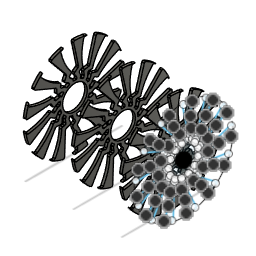
knobs + spokes v4 (Autodesk Fusion 360 archive; units mm, degrees)
design "spoke support"
Autodesk Fusion 360 part; units mm, degrees
sketch "Sketch1" plane through (0, 0, 0) normal (1, 0, 0) x (0, 0, -1)
  circle A0 centre (0, 0) radius 5
  circle A1 centre (0, 0) radius 20 construction
  circle A2 centre (0, 0) radius 6
  line L0 (-0.021, 20) -> (-0.0893, 19.9864)
  line L1 (-0.481, 19.3928) -> (1.4345, 10.3121)
  line L2 (1.2453, 9.8089) -> (-0.1, 8.8)
  line L3 (-0.2, 8.1) -> (0.71, 6.8867)
  line L4 (0.75, 6.7667) -> (0.75, 5.9529)
  arc A3 (-0.0893, 19.9864) -> (-0.481, 19.3928) centre (0.0083, 19.496) ccw
  arc A4 (1.2453, 9.8089) -> (1.4345, 10.3121) centre (0.9453, 10.2089) ccw
  arc A5 (-0.1, 8.8) -> (-0.2, 8.1) centre (0.2, 8.4) ccw
  arc A6 (0.75, 6.7667) -> (0.71, 6.8867) centre (0.55, 6.7667) ccw
  line L5 (4.9442, 19.3792) -> (4.0475, 19.3979)
  arc A7 (4.0475, 19.3979) -> (3.5372, 18.9052) centre (4.0371, 18.898) ccw
  arc A8 (2.9152, 8.8921) -> (3.1386, 9.6333) centre (2.7238, 9.3541) ccw
  line L6 (2.9152, 8.8921) -> (2.0875, 8.5494)
  arc A9 (2.0875, 8.5494) -> (1.8169, 7.8961) centre (2.2789, 8.0874) ccw
  line L7 (1.8169, 7.8961) -> (2.3972, 6.4949)
  arc A10 (2.4062, 6.3687) -> (2.3972, 6.4949) centre (2.2124, 6.4184) ccw
  line L8 (2.4062, 6.3687) -> (2.2042, 5.5805)
  spline S0 degree 5 poles (3.5372, 18.9052) (3.4914, 18.7092) (3.403, 18.318) (3.2802, 17.7339) (3.1365, 16.9608) (2.9923, 16.0043) (2.887, 15.0588) (2.8238, 14.1251) (2.8051, 13.2038) (2.8293, 12.2946) (2.8936, 11.3966) (2.9744, 10.6864) (3.0506, 10.1582) (3.1082, 9.8079) (3.1386, 9.6333) knots 0 0 0 0 0 0 0.1 0.2 0.3 0.4 0.5 0.6 0.7 0.8 0.9 1 1 1 1 1 1
  arc A11 (4.9442, 19.3792) -> (-0.021, 20) centre (0, 0) ccw
  line L9 (-2.4805, 6.3401) -> (-2.1024, 5.6196)
  arc A12 (-2.4805, 6.3401) -> (-2.5717, 6.4278) centre (-2.6576, 6.2472) ccw
  line L10 (-3.9413, 7.0792) -> (-2.5717, 6.4278)
  arc A13 (-4.1781, 7.7455) -> (-3.9413, 7.0792) centre (-3.7265, 7.5308) ccw
  line L11 (-3.4558, 9.264) -> (-4.1781, 7.7455)
  arc A14 (-3.4558, 9.264) -> (-3.5221, 9.7975) centre (-3.9073, 9.4788) ccw
  line L12 (-9.4382, 16.948) -> (-3.5221, 9.7975)
  arc A15 (-9.3672, 17.6555) -> (-9.4382, 16.948) centre (-9.0529, 17.2667) ccw
  line L13 (-9.313, 17.6994) -> (-9.3672, 17.6555)
  arc A16 (-4.6281, 19.4571) -> (-9.313, 17.6994) centre (0, 0) ccw
  line L14 (-4.6281, 19.4571) -> (-5.4307, 19.057)
  arc A17 (-5.4307, 19.057) -> (-5.6537, 18.3836) centre (-5.2076, 18.6095) ccw
  arc A18 (-1.5511, 9.2283) -> (-1.6977, 9.9884) centre (-1.9352, 9.5485) ccw
  line L15 (-1.5511, 9.2283) -> (-2.1247, 8.5402)
  arc A19 (-2.1247, 8.5402) -> (-2.0607, 7.836) centre (-1.7406, 8.2201) ccw
  line L16 (-2.0607, 7.836) -> (-0.8957, 6.865)
  arc A20 (-0.8291, 6.7574) -> (-0.8957, 6.865) centre (-1.0237, 6.7114) ccw
  line L17 (-0.8291, 6.7574) -> (-0.6417, 5.9656)
  spline S1 degree 5 poles (-5.6537, 18.3836) (-5.6031, 18.1887) (-5.4996, 17.8012) (-5.3369, 17.227) (-5.1049, 16.4756) (-4.788, 15.5617) (-4.4419, 14.6755) (-4.0639, 13.8194) (-3.6523, 12.9949) (-3.2083, 12.2011) (-2.7341, 11.4359) (-2.3325, 10.8446) (-2.0196, 10.4123) (-1.8058, 10.1289) (-1.6977, 9.9884) knots 0 0 0 0 0 0 0.1 0.2 0.3 0.4 0.5 0.6 0.7 0.8 0.9 1 1 1 1 1 1
  line L18 (-5.1428, 4.4611) -> (-4.4731, 3.9989)
  arc A21 (-5.1428, 4.4611) -> (-5.2643, 4.4964) centre (-5.2564, 4.2965) ccw
  line L19 (-6.7797, 4.4367) -> (-5.2643, 4.4964)
  arc A22 (-7.299, 4.9167) -> (-6.7797, 4.4367) centre (-6.7994, 4.9363) ccw
  line L20 (-7.3652, 6.5969) -> (-7.299, 4.9167)
  arc A23 (-7.3652, 6.5969) -> (-7.6718, 7.0385) centre (-7.8648, 6.5772) ccw
  line L21 (-16.2332, 10.6205) -> (-7.6718, 7.0385)
  arc A24 (-16.4992, 11.28) -> (-16.2332, 10.6205) centre (-16.0402, 11.0818) ccw
  line L22 (-16.4716, 11.344) -> (-16.4992, 11.28)
  arc A25 (-13.1402, 15.0777) -> (-16.4716, 11.344) centre (0, 0) ccw
  line L23 (-13.1402, 15.0777) -> (-13.6649, 14.3503)
  arc A26 (-13.6649, 14.3503) -> (-13.5494, 13.6505) centre (-13.2594, 14.0578) ccw
  arc A27 (-5.6621, 7.4504) -> (-6.1451, 8.0554) centre (-6.1509, 7.5554) ccw
  line L24 (-5.6621, 7.4504) -> (-5.8501, 6.5746)
  arc A28 (-5.8501, 6.5746) -> (-5.4662, 5.9808) centre (-5.3613, 6.4696) ccw
  line L25 (-5.4662, 5.9808) -> (-3.9834, 5.6624)
  arc A29 (-3.8745, 5.5981) -> (-3.9834, 5.6624) centre (-4.0254, 5.4669) ccw
  line L26 (-3.8745, 5.5981) -> (-3.3405, 4.9841)
  spline S2 degree 5 poles (-13.5494, 13.6505) (-13.414, 13.5014) (-13.1423, 13.2064) (-12.7314, 12.7736) (-12.1768, 12.2161) (-11.4715, 11.5541) (-10.7531, 10.9303) (-10.0206, 10.3479) (-9.273, 9.8091) (-8.511, 9.3126) (-7.7354, 8.8553) (-7.1051, 8.5185) (-6.6271, 8.2811) (-6.3061, 8.1295) (-6.1451, 8.0554) knots 0 0 0 0 0 0 0.1 0.2 0.3 0.4 0.5 0.6 0.7 0.8 0.9 1 1 1 1 1 1
  line L27 (-6.6269, 1.5602) -> (-5.8191, 1.4621)
  arc A30 (-6.6269, 1.5602) -> (-6.7509, 1.5349) centre (-6.651, 1.3616) ccw
  line L28 (-8.065, 0.7778) -> (-6.7509, 1.5349)
  arc A31 (-8.7478, 0.9615) -> (-8.065, 0.7778) centre (-8.3146, 1.2111) ccw
  line L29 (-9.5873, 2.4185) -> (-8.7478, 0.9615)
  arc A32 (-9.5873, 2.4185) -> (-10.064, 2.667) centre (-10.0205, 2.1689) ccw
  line L30 (-19.3094, 1.8601) -> (-10.064, 2.667)
  arc A33 (-19.8514, 2.3204) -> (-19.3094, 1.8601) centre (-19.3529, 2.3582) ccw
  line L31 (-19.8567, 2.3899) -> (-19.8514, 2.3204)
  arc A34 (-18.642, 7.2441) -> (-19.8567, 2.3899) centre (0, 0) ccw
  line L32 (-18.642, 7.2441) -> (-18.7686, 6.3562)
  arc A35 (-18.7686, 6.3562) -> (-18.341, 5.7902) centre (-18.2736, 6.2856) ccw
  arc A36 (-8.4759, 3.9657) -> (-9.1847, 4.2769) centre (-8.9576, 3.8315) ccw
  line L33 (-8.4759, 3.9657) -> (-8.2354, 3.1028)
  arc A37 (-8.2354, 3.1028) -> (-7.6195, 2.7554) centre (-7.7538, 3.2371) ccw
  line L34 (-7.6195, 2.7554) -> (-6.1586, 3.1626)
  arc A38 (-6.0323, 3.1563) -> (-6.1586, 3.1626) centre (-6.1049, 2.97) ccw
  line L35 (-6.0323, 3.1563) -> (-5.2741, 2.8608)
  spline S3 degree 5 poles (-18.341, 5.7902) (-18.1519, 5.721) (-17.7742, 5.5862) (-17.2092, 5.3939) (-16.4591, 5.158) (-15.527, 4.8996) (-14.601, 4.6811) (-13.6817, 4.5058) (-12.7694, 4.3761) (-11.8639, 4.2906) (-10.9647, 4.2462) (-10.25, 4.2408) (-9.7164, 4.2528) (-9.3617, 4.2677) (-9.1847, 4.2769) knots 0 0 0 0 0 0 0.1 0.2 0.3 0.4 0.5 0.6 0.7 0.8 0.9 1 1 1 1 1 1
  line L36 (-6.5929, -1.6982) -> (-5.832, -1.4097)
  arc A39 (-6.5929, -1.6982) -> (-6.6909, -1.7782) centre (-6.522, -1.8852) ccw
  line L37 (-7.5027, -3.0593) -> (-6.6909, -1.7782)
  arc A40 (-8.1927, -3.214) -> (-7.5027, -3.0593) centre (-7.925, -2.7916) ccw
  line L38 (-9.613, -2.3139) -> (-8.1927, -3.214)
  arc A41 (-9.613, -2.3139) -> (-10.1506, -2.3154) centre (-9.8807, -2.7363) ccw
  line L39 (-17.962, -7.3265) -> (-10.1506, -2.3154)
  arc A42 (-18.6559, -7.1708) -> (-17.962, -7.3265) centre (-18.232, -6.9056) ccw
  line L40 (-18.6929, -7.1117) -> (-18.6559, -7.1708)
  arc A43 (-19.8731, -2.2491) -> (-18.6929, -7.1117) centre (0, 0) ccw
  line L41 (-19.8731, -2.2491) -> (-19.5726, -3.0941)
  arc A44 (-19.5726, -3.0941) -> (-18.931, -3.3966) centre (-19.1015, -2.9265) ccw
  arc A45 (-9.348, -0.4275) -> (-10.1202, -0.4813) centre (-9.7121, -0.7702) ccw
  line L42 (-9.348, -0.4275) -> (-8.734, -1.0798)
  arc A46 (-8.734, -1.0798) -> (-8.0273, -1.1012) centre (-8.37, -0.7371) ccw
  line L43 (-8.0273, -1.1012) -> (-6.9229, -0.0617)
  arc A47 (-6.8081, -0.0086) -> (-6.9229, -0.0617) centre (-6.7858, -0.2073) ccw
  line L44 (-6.8081, -0.0086) -> (-5.9994, 0.0821)
  spline S4 degree 5 poles (-18.931, -3.3966) (-18.7314, -3.3699) (-18.3343, -3.3138) (-17.7447, -3.2215) (-16.9708, -3.0817) (-16.0254, -2.8774) (-15.1039, -2.6405) (-14.2085, -2.3685) (-13.3404, -2.0593) (-12.4989, -1.7142) (-11.682, -1.3357) (-11.0467, -1.0083) (-10.5798, -0.7498) (-10.2727, -0.5718) (-10.1202, -0.4813) knots 0 0 0 0 0 0 0.1 0.2 0.3 0.4 0.5 0.6 0.7 0.8 0.9 1 1 1 1 1 1
  line L45 (-5.0485, -4.5676) -> (-4.5089, -3.9585)
  arc A48 (-5.0485, -4.5676) -> (-5.0981, -4.6839) centre (-4.8988, -4.7002) ccw
  line L46 (-5.2216, -6.1955) -> (-5.0981, -4.6839)
  arc A49 (-5.7606, -6.6532) -> (-5.2216, -6.1955) centre (-5.7199, -6.1548) ccw
  line L47 (-7.4366, -6.5163) -> (-5.7606, -6.6532)
  arc A50 (-7.4366, -6.5163) -> (-7.9119, -6.7675) centre (-7.4773, -7.0146) ccw
  line L48 (-12.4998, -14.8347) -> (-7.9119, -6.7675)
  arc A51 (-13.1865, -15.0193) -> (-12.4998, -14.8347) centre (-12.9344, -14.5875) ccw
  line L49 (-13.2468, -14.9841) -> (-13.1865, -15.0193)
  arc A52 (-16.5516, -11.227) -> (-13.2468, -14.9841) centre (0, 0) ccw
  line L50 (-16.5516, -11.227) -> (-15.8928, -11.8355)
  arc A53 (-15.8928, -11.8355) -> (-15.1841, -11.8052) centre (-15.5535, -11.4682) ccw
  arc A54 (-8.0786, -4.7227) -> (-8.7373, -5.1293) centre (-8.2417, -5.1954) ccw
  line L51 (-8.0786, -4.7227) -> (-7.2318, -5.015)
  arc A55 (-7.2318, -5.015) -> (-6.596, -4.7055) centre (-7.0687, -4.5424) ccw
  line L52 (-6.596, -4.7055) -> (-6.1013, -3.2718)
  arc A56 (-6.0243, -3.1715) -> (-6.1013, -3.2718) centre (-5.9122, -3.3371) ccw
  line L53 (-6.0243, -3.1715) -> (-5.3504, -2.7154)
  spline S5 degree 5 poles (-15.1841, -11.8052) (-15.0198, -11.6888) (-14.6942, -11.4546) (-14.215, -11.0989) (-13.5948, -10.6155) (-12.8526, -9.9952) (-12.1468, -9.3572) (-11.4803, -8.7002) (-10.8553, -8.0231) (-10.2706, -7.3264) (-9.7232, -6.6117) (-9.3128, -6.0265) (-9.0195, -5.5806) (-8.8303, -5.2802) (-8.7373, -5.1293) knots 0 0 0 0 0 0 0.1 0.2 0.3 0.4 0.5 0.6 0.7 0.8 0.9 1 1 1 1 1 1
  line L54 (-2.3476, -6.3906) -> (-2.1528, -5.6005)
  arc A57 (-2.3476, -6.3906) -> (-2.3375, -6.5166) centre (-2.1534, -6.4384) ccw
  line L55 (-1.7443, -7.9124) -> (-2.3375, -6.5166)
  arc A58 (-2.0089, -8.5682) -> (-1.7443, -7.9124) centre (-2.2045, -8.108) ccw
  line L56 (-3.5565, -9.2258) -> (-2.0089, -8.5682)
  arc A59 (-3.5565, -9.2258) -> (-3.8606, -9.6691) centre (-3.3609, -9.686) ccw
  line L57 (-4.174, -18.9444) -> (-3.8606, -9.6691)
  arc A60 (-4.6963, -19.427) -> (-4.174, -18.9444) centre (-4.6737, -18.9275) ccw
  line L58 (-4.766, -19.4238) -> (-4.6963, -19.427)
  arc A61 (-9.4383, -17.6329) -> (-4.766, -19.4238) centre (0, 0) ccw
  line L59 (-9.4383, -17.6329) -> (-8.5721, -17.8656)
  arc A62 (-8.5721, -17.8656) -> (-7.9587, -17.5094) centre (-8.4424, -17.3827) ccw
  arc A63 (-4.9585, -7.9361) -> (-5.3528, -8.6022) centre (-4.8833, -8.4304) ccw
  line L60 (-4.9585, -7.9361) -> (-4.0729, -7.8014)
  arc A64 (-4.0729, -7.8014) -> (-3.6538, -7.2318) centre (-4.1481, -7.307) ccw
  line L61 (-3.6538, -7.2318) -> (-3.8819, -5.7325)
  arc A65 (-3.8604, -5.6078) -> (-3.8819, -5.7325) centre (-3.6842, -5.7024) ccw
  line L62 (-3.8604, -5.6078) -> (-3.4756, -4.8908)
  spline S6 degree 5 poles (-7.9587, -17.5094) (-7.8673, -17.33) (-7.6879, -16.9713) (-7.4289, -16.4336) (-7.1043, -15.7173) (-6.7354, -14.8232) (-6.4069, -13.9303) (-6.1221, -13.0388) (-5.8834, -12.1488) (-5.6894, -11.2602) (-5.5369, -10.3729) (-5.4454, -9.6641) (-5.393, -9.1329) (-5.365, -8.7791) (-5.3528, -8.6022) knots 0 0 0 0 0 0 0.1 0.2 0.3 0.4 0.5 0.6 0.7 0.8 0.9 1 1 1 1 1 1
  line L63 (0.8912, -6.7495) -> (0.6964, -5.9594)
  arc A66 (0.8912, -6.7495) -> (0.9587, -6.8565) centre (1.0854, -6.7017) ccw
  line L64 (2.1326, -7.8167) -> (0.9587, -6.8565)
  arc A67 (2.203, -8.5203) -> (2.1326, -7.8167) centre (1.816, -8.2037) ccw
  line L65 (1.1383, -9.8219) -> (2.203, -8.5203)
  arc A68 (1.1383, -9.8219) -> (1.075, -10.3557) centre (1.5254, -10.1384) ccw
  line L66 (5.108, -18.7142) -> (1.075, -10.3557)
  arc A69 (4.8698, -19.3842) -> (5.108, -18.7142) centre (4.6577, -18.9315) ccw
  line L67 (4.8067, -19.4138) -> (4.8698, -19.3842)
  arc A70 (-0.1628, -19.9993) -> (4.8067, -19.4138) centre (0, 0) ccw
  line L68 (-0.1628, -19.9993) -> (0.7123, -19.8029)
  arc A71 (0.7123, -19.8029) -> (1.0899, -19.2024) centre (0.6028, -19.315) ccw
  arc A72 (-0.7024, -9.3314) -> (-0.742, -10.1045) centre (-0.4061, -9.7341) ccw
  line L69 (-0.7024, -9.3314) -> (0.0191, -8.8005)
  arc A73 (0.0191, -8.8005) -> (0.1255, -8.1015) centre (-0.2772, -8.3978) ccw
  line L70 (0.1255, -8.1015) -> (-0.7732, -6.8799)
  arc A74 (-0.8121, -6.7595) -> (-0.7732, -6.8799) centre (-0.6121, -6.7613) ccw
  line L71 (-0.8121, -6.7595) -> (-0.8047, -5.9458)
  spline S7 degree 5 poles (1.0899, -19.2024) (1.0875, -19.0011) (1.0797, -18.6001) (1.0591, -18.0036) (1.0137, -17.2185) (0.9247, -16.2554) (0.8007, -15.3121) (0.6386, -14.3904) (0.4363, -13.4914) (0.1952, -12.6144) (-0.0821, -11.7579) (-0.3306, -11.0877) (-0.5309, -10.593) (-0.6707, -10.2667) (-0.742, -10.1045) knots 0 0 0 0 0 0 0.1 0.2 0.3 0.4 0.5 0.6 0.7 0.8 0.9 1 1 1 1 1 1
  line L72 (3.9257, -5.5623) -> (3.3861, -4.9532)
  arc A75 (3.9257, -5.5623) -> (4.0353, -5.6256) centre (4.0755, -5.4296) ccw
  line L73 (5.5209, -5.9303) -> (4.0353, -5.6256)
  arc A76 (5.9103, -6.5206) -> (5.5209, -5.9303) centre (5.4205, -6.4201) ccw
  line L74 (5.5724, -8.1678) -> (5.9103, -6.5206)
  arc A77 (5.5724, -8.1678) -> (5.7644, -8.6699) centre (6.0622, -8.2683) ccw
  line L75 (13.2198, -14.1968) -> (5.7644, -8.6699)
  arc A78 (13.3203, -14.9008) -> (13.2198, -14.1968) centre (12.922, -14.5984) ccw
  line L76 (13.2781, -14.9563) -> (13.3203, -14.9008)
  arc A79 (9.15, -17.7842) -> (13.2781, -14.9563) centre (0, 0) ccw
  line L77 (9.15, -17.7842) -> (9.8336, -17.2035)
  arc A80 (9.8336, -17.2035) -> (9.8889, -16.4964) centre (9.5098, -16.8225) ccw
  arc A81 (3.7145, -8.589) -> (4.0387, -9.2919) centre (4.1641, -8.8079) ccw
  line L78 (3.7145, -8.589) -> (4.1067, -7.7836)
  arc A82 (4.1067, -7.7836) -> (3.8761, -7.1151) centre (3.6572, -7.5647) ccw
  line L79 (3.8761, -7.1151) -> (2.5126, -6.4511)
  arc A83 (2.4222, -6.3626) -> (2.5126, -6.4511) centre (2.6001, -6.2713) ccw
  line L80 (2.4222, -6.3626) -> (2.0507, -5.6387)
  spline S8 degree 5 poles (9.8889, -16.4964) (9.7932, -16.3192) (9.5999, -15.9678) (9.3045, -15.4492) (8.8994, -14.7752) (8.3731, -13.9637) (7.8249, -13.1861) (7.253, -12.4453) (6.6561, -11.7433) (6.035, -11.0788) (5.3914, -10.4492) (4.86, -9.9713) (4.4527, -9.6264) (4.1774, -9.4024) (4.0387, -9.2919) knots 0 0 0 0 0 0 0.1 0.2 0.3 0.4 0.5 0.6 0.7 0.8 0.9 1 1 1 1 1 1
  line L81 (6.061, -3.1008) -> (5.3001, -2.8122)
  arc A84 (6.061, -3.1008) -> (6.1874, -3.1059) centre (6.1319, -2.9138) ccw
  line L82 (7.6445, -2.6853) -> (6.1874, -3.1059)
  arc A85 (8.2636, -3.027) -> (7.6445, -2.6853) centre (7.7832, -3.1657) ccw
  line L83 (8.7299, -4.6426) -> (8.2636, -3.027)
  arc A86 (8.7299, -4.6426) -> (9.1333, -4.998) centre (9.2103, -4.5039) ccw
  line L84 (18.3031, -6.4271) -> (9.1333, -4.998)
  arc A87 (18.7193, -7.0037) -> (18.3031, -6.4271) centre (18.2261, -6.9211) ccw
  line L85 (18.7077, -7.0725) -> (18.7193, -7.0037)
  arc A88 (16.3667, -11.4949) -> (18.7077, -7.0725) centre (0, 0) ccw
  line L86 (16.3667, -11.4949) -> (16.7021, -10.6631)
  arc A89 (16.7021, -10.6631) -> (16.4224, -10.0112) centre (16.2383, -10.4761) ccw
  arc A90 (7.2806, -5.8789) -> (7.8943, -6.3507) centre (7.7803, -5.8638) ccw
  line L87 (7.2806, -5.8789) -> (7.2535, -4.9835)
  arc A91 (7.2535, -4.9835) -> (6.7387, -4.4988) centre (6.7538, -4.9986) ccw
  line L88 (6.7387, -4.4988) -> (5.2228, -4.5446)
  arc A92 (5.1016, -4.5082) -> (5.2228, -4.5446) centre (5.2167, -4.3447) ccw
  line L89 (5.1016, -4.5082) -> (4.4362, -4.0398)
  spline S9 degree 5 poles (16.4224, -10.0112) (16.2553, -9.8988) (15.9209, -9.6775) (15.4183, -9.3556) (14.7464, -8.947) (13.9032, -8.4731) (13.0565, -8.0393) (12.2058, -7.6492) (11.351, -7.3049) (10.4923, -7.0052) (9.6299, -6.7468) (8.9372, -6.5706) (8.4163, -6.4545) (8.0684, -6.3841) (7.8943, -6.3507) knots 0 0 0 0 0 0 0.1 0.2 0.3 0.4 0.5 0.6 0.7 0.8 0.9 1 1 1 1 1 1
  line L90 (6.8077, 0.0711) -> (5.9999, -0.027)
  arc A93 (6.8077, 0.0711) -> (6.922, 0.1253) centre (6.7836, 0.2696) ccw
  line L91 (8.0168, 1.1749) -> (6.922, 0.1253)
  arc A94 (8.7238, 1.16) -> (8.0168, 1.1749) centre (8.3628, 0.8139) ccw
  line L92 (9.8875, -0.0538) -> (8.7238, 1.16)
  arc A95 (9.8875, -0.0538) -> (10.4098, -0.1811) centre (10.2484, 0.2922) ccw
  line L93 (19.1934, 2.815) -> (10.4098, -0.1811)
  arc A96 (19.8299, 2.4978) -> (19.1934, 2.815) centre (19.3548, 2.3418) ccw
  line L94 (19.8516, 2.4315) -> (19.8299, 2.4978)
  arc A97 (19.8339, -2.5722) -> (19.8516, 2.4315) centre (0, 0) ccw
  line L95 (19.8339, -2.5722) -> (19.7443, -1.6799)
  arc A98 (19.7443, -1.6799) -> (19.1938, -1.2326) centre (19.2468, -1.7298) ccw
  arc A99 (9.1787, -1.8221) -> (9.9413, -1.9546) centre (9.6142, -1.5765) ccw
  line L96 (9.1787, -1.8221) -> (8.7386, -1.0418)
  arc A100 (8.7386, -1.0418) -> (8.0575, -0.8519) centre (8.3031, -1.2874) ccw
  line L97 (8.0575, -0.8519) -> (6.7365, -1.5969)
  arc A101 (6.6123, -1.621) -> (6.7365, -1.5969) centre (6.6382, -1.4227) ccw
  line L98 (6.6123, -1.621) -> (5.8055, -1.5155)
  spline S10 degree 5 poles (19.1938, -1.2326) (18.9936, -1.2108) (18.5946, -1.1702) (18, -1.1187) (17.2152, -1.0692) (16.2483, -1.0414) (15.297, -1.0508) (14.3624, -1.1007) (13.4456, -1.1931) (12.546, -1.3268) (11.6622, -1.4988) (10.967, -1.6646) (10.4518, -1.8039) (10.111, -1.9033) (9.9413, -1.9546) knots 0 0 0 0 0 0 0.1 0.2 0.3 0.4 0.5 0.6 0.7 0.8 0.9 1 1 1 1 1 1
  line L99 (5.9949, 3.2267) -> (5.3252, 2.7644)
  arc A102 (5.9949, 3.2267) -> (6.0709, 3.3278) centre (5.8813, 3.3913) ccw
  line L100 (6.5525, 4.7659) -> (6.0709, 3.3278)
  arc A103 (7.1854, 5.0812) -> (6.5525, 4.7659) centre (7.0267, 4.6071) ccw
  line L101 (8.7799, 4.5472) -> (7.1854, 5.0812)
  arc A104 (8.7799, 4.5472) -> (9.3016, 4.6774) centre (8.9387, 5.0214) ccw
  line L102 (15.6867, 11.4122) -> (9.3016, 4.6774)
  arc A105 (16.3977, 11.4271) -> (15.6867, 11.4122) centre (16.0496, 11.0682) ccw
  line L103 (16.4478, 11.3785) -> (16.3977, 11.4271)
  arc A106 (18.7574, 6.9397) -> (16.4478, 11.3785) centre (0, 0) ccw
  line L104 (18.7574, 6.9397) -> (18.2634, 7.6882)
  arc A107 (18.2634, 7.6882) -> (17.5681, 7.8283) centre (17.8461, 7.4128) ccw
  arc A108 (8.9741, 2.6522) -> (9.711, 2.8893) centre (9.2456, 3.072) ccw
  line L105 (8.9741, 2.6522) -> (8.2218, 3.1386)
  arc A109 (8.2218, 3.1386) -> (7.5305, 2.9902) centre (7.9503, 2.7187) ccw
  line L106 (7.5305, 2.9902) -> (6.707, 1.7166)
  arc A110 (6.6082, 1.6376) -> (6.707, 1.7166) centre (6.539, 1.8252) ccw
  line L107 (6.6082, 1.6376) -> (5.8448, 1.356)
  spline S11 degree 5 poles (17.5681, 7.8283) (17.3807, 7.7547) (17.0085, 7.6052) (16.4581, 7.3745) (15.7402, 7.0536) (14.8711, 6.6289) (14.0331, 6.1784) (13.2288, 5.7) (12.4599, 5.1921) (11.7255, 4.6556) (11.0229, 4.0926) (10.4844, 3.6227) (10.0929, 3.2599) (9.8374, 3.0136) (9.711, 2.8893) knots 0 0 0 0 0 0 0.1 0.2 0.3 0.4 0.5 0.6 0.7 0.8 0.9 1 1 1 1 1 1
  line L108 (3.8087, 5.643) -> (3.4306, 4.9225)
  arc A111 (3.8087, 5.643) -> (3.8291, 5.7679) centre (3.6316, 5.736) ccw
  line L109 (3.5872, 7.2651) -> (3.8291, 5.7679)
  arc A112 (4.001, 7.8384) -> (3.5872, 7.2651) centre (4.0808, 7.3448) ccw
  line L110 (5.661, 8.1066) -> (4.001, 7.8384)
  arc A113 (5.661, 8.1066) -> (6.0624, 8.4642) centre (5.5813, 8.6002) ccw
  line L111 (8.5864, 17.395) -> (6.0624, 8.4642)
  arc A114 (9.209, 17.7386) -> (8.5864, 17.395) centre (9.0676, 17.259) ccw
  line L112 (9.2759, 17.7188) -> (9.209, 17.7386)
  arc A115 (13.3838, 14.8618) -> (9.2759, 17.7188) centre (0, 0) ccw
  line L113 (13.3838, 14.8618) -> (12.5986, 15.295)
  arc A116 (12.5986, 15.295) -> (11.9177, 15.0959) centre (12.357, 14.8572) ccw
  arc A117 (6.7136, 6.5188) -> (7.2559, 7.0712) centre (6.7589, 7.0168) ccw
  line L114 (6.7136, 6.5188) -> (5.8215, 6.6)
  arc A118 (5.8215, 6.6) -> (5.2783, 6.1473) centre (5.7762, 6.102) ccw
  line L115 (5.2783, 6.1473) -> (5.141, 4.6369)
  arc A119 (5.0903, 4.521) -> (5.141, 4.6369) centre (4.9418, 4.655) ccw
  line L116 (5.0903, 4.521) -> (4.5451, 3.9169)
  spline S12 degree 5 poles (11.9177, 15.0959) (11.786, 14.9436) (11.526, 14.6383) (11.1458, 14.1782) (10.6593, 13.5605) (10.0871, 12.7806) (9.5545, 11.9922) (9.0646, 11.1948) (8.6199, 10.3878) (8.2188, 9.5714) (7.8584, 8.7464) (7.5999, 8.0801) (7.4219, 7.5769) (7.3101, 7.24) (7.2559, 7.0712) knots 0 0 0 0 0 0 0.1 0.2 0.3 0.4 0.5 0.6 0.7 0.8 0.9 1 1 1 1 1 1
  point P0 (2.8304, 14.0199)
  point P1 (-4.0091, 13.7293)
  point P2 (-9.9303, 10.2936)
  point P3 (-13.5765, 4.4997)
  point P4 (-14.1125, -2.325)
  point P5 (-11.4155, -8.6171)
  point P6 (-6.1033, -12.9351)
  point P7 (0.607, -14.2898)
  point P8 (7.1783, -12.3709)
  point P9 (12.1051, -7.618)
  point P10 (14.2588, -1.1199)
  point P11 (13.146, 5.6348)
  point P12 (9.0216, 11.0986)
  dimension "d1" = 10
  dimension "d2" = 40
  dimension "d3" = 12
  dimension "d4" = 0.5
  dimension "d5" = 0.5
  dimension "d6" = 0.5
  dimension "d7" = 0.2
  dimension "d8" = 0.5
  dimension "d9" = 0.5
  dimension "d10" = 0.5
  dimension "d11" = 0.2
  dimension "d12" = 40
  dimension "d14" = 360
  constraint coincident A0.centre A1.centre
  constraint concentric A0 A2
  constraint coincident A1 L0.start
  constraint perpendicular L2 L3
  constraint coincident A2 L4.end
  constraint vertical L4
  constraint tangent L0 A3
  constraint tangent L1 A3
  constraint tangent L1 A4
  constraint tangent L2 A4
  constraint tangent L2 A5
  constraint tangent L3 A5
  constraint tangent L3 A6
  constraint tangent L4 A6
  constraint perpendicular L6 L7
  constraint tangent L5 A7
  constraint tangent A8 L6
  constraint tangent L6 A9
  constraint tangent A9 L7
  constraint tangent L7 A10
  constraint tangent A10 L8
  constraint coincident A1 L5.start
  constraint coincident A2 L8.end
  measures "d1" diameter of A0
  measures "d2" diameter of A1
  measures "d3" diameter of A2
  measures "d4" radius of A3
  measures "d5" radius of A4
  measures "d6" radius of A5
  measures "d7" radius of A6
  measures "d8" radius of A7
  measures "d9" radius of A8
  measures "d10" radius of A9
  measures "d11" radius of A10
  measures "d12" diameter of A11
extrude "Extrude1" add sketch "Sketch1" against normal blind 50 makes body 1
sketch "Sketch2" plane through (0, 0, 0) normal (0, 0, 1) x (1, 0, 0)
  line L0 (-24.5, -20) -> (-25.5, -20)
  line L1 (-25.5, -20) -> (-25.5, 20)
  line L2 (-25.5, 20) -> (-24.5, 20)
  line L3 (-24.5, 20) -> (-24.5, -20)
  line L4 (-24.5, -20) -> (-25.5, 20) construction
  line L5 (-25.5, -20) -> (-24.5, 20) construction
  line L6 (0, -20) -> (-50, -20)
  line L7 (-50, -20) -> (-50, 20)
  line L8 (-50, 20) -> (0, 20)
  line L9 (0, 20) -> (0, -20)
  line L10 (0, -20) -> (-50, 20) construction
  line L11 (-50, -20) -> (0, 20) construction
  line L12 (-5, -20) -> (-45, -20)
  line L13 (-45, -20) -> (-45, 20)
  line L14 (-45, 20) -> (-5, 20)
  line L15 (-5, 20) -> (-5, -20)
  line L16 (-5, -20) -> (-45, 20) construction
  line L17 (-45, -20) -> (-5, 20) construction
  line L18 (-6, -20) -> (-44, -20)
  line L19 (-44, -20) -> (-44, 20)
  line L20 (-44, 20) -> (-6, 20)
  line L21 (-6, 20) -> (-6, -20)
  line L22 (-6, -20) -> (-44, 20) construction
  line L23 (-44, -20) -> (-6, 20) construction
  point P0 (-25, 0)
  point P1 (-25, 0)
  point P2 (-25, 0)
  point P3 (-25, 0)
  dimension "d17" = 1
  dimension "d18" = 40
  constraint horizontal L0
  constraint perpendicular L0 L1
  constraint parallel L0 L2
  constraint parallel L1 L3
  constraint coincident L4 P3
  constraint coincident L5 P3
  constraint horizontal L6
  constraint perpendicular L6 L7
  constraint parallel L6 L8
  constraint parallel L7 L9
  constraint coincident L10 P3
  constraint coincident L11 P3
  constraint coincident P3 P2
  constraint horizontal L12
  constraint perpendicular L12 L13
  constraint parallel L12 L14
  constraint parallel L13 L15
  constraint coincident L16 P3
  constraint coincident L17 P3
  constraint coincident L6 L12.start
  constraint horizontal L18
  constraint perpendicular L18 L19
  constraint parallel L18 L20
  constraint parallel L19 L21
  constraint coincident L22 P3
  constraint coincident L23 P3
  constraint coincident L6 L18.start
  measures "d17" distance of L1.end L2.end
  measures "d18" distance of L0.end L1.end
extrude "Extrude2" cut sketch "Sketch2" along normal mid plane 42 contours L3 L6 L8 L12 L14 L18 L20 L21 | L1 L6 L8 L12 L14 L18 L19 L20 | L6 L8 L9 L15 | L6 L7 L8 L13 bodies 1 makes body 2 at (-24.5, 9.0711, 10.9258) makes body 3 at (-45, 2.9546, 13.8899)
